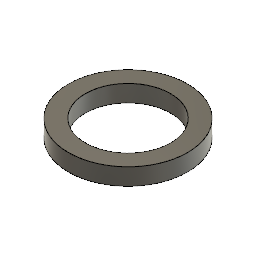
5mm_XY_Idler_Mount v15 (Autodesk Fusion 360 archive; units mm, degrees)
design "Spacer_5x7x1"
Autodesk Fusion 360 part; units mm, degrees
sketch "Sketch1" plane through (0, 0, 0) normal (0, 1, 0) x (1, 0, 0)
  circle A0 centre (0, 0) radius 2.5
  circle A1 centre (0, 0) radius 3.5
  dimension "d1" = 5
  dimension "d2" = 7
  constraint coincident A0.centre A1.centre
  constraint concentric A0 A1
  measures "d1" diameter of A0
  measures "d2" diameter of A1
extrude "Extrude2" add sketch "Sketch1" along normal blind 1

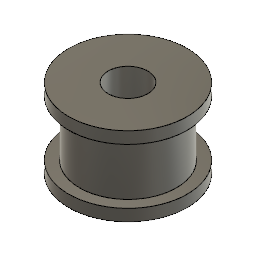
design "LDO_20T_5mm_pulley"
Autodesk Fusion 360 part; units mm, degrees
sketch "Sketch1" plane through (0, 0, 0) normal (0, 1, 0) x (1, 0, 0)
  circle A0 centre (0, 0) radius 2.5
  circle A1 centre (0, 0) radius 6.125
  circle A2 centre (0, 0) radius 7.5
  dimension "d1" = 5
  dimension "d2" = 12.25
  dimension "d3" = 15
  constraint coincident A0.centre A1.centre
  constraint concentric A0 A2
  measures "d1" diameter of A0
  measures "d2" diameter of A1
  measures "d3" diameter of A2
extrude "Extrude1" add sketch "Sketch1" along normal blind 10 contours A1
extrude "Extrude2" add sketch "Sketch1" along normal blind 1.5 contours A2
extrude "Extrude3" add sketch "Sketch1" against normal blind 1.5 from surface at 10 contours A2
